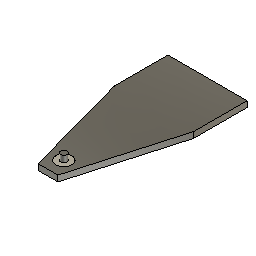
Top Mounting Plate v10 (Autodesk Fusion 360 design; units mm, degrees)
Autodesk Fusion 360 part; units mm, degrees
note: some values were not read from the file. Set by a fixed rule: which sketch regions a step uses.
sketch "Sketch1" plane through (0, 0, 0) normal (0, 0, 1) x (1, 0, 0)
  line L0 (0, 0) -> (-127, 0)
  line L1 (-127, 0) -> (-127, -85.725)
  line L2 (-127, -85.725) -> (0, -85.725)
  line L3 (0, -85.725) -> (0, 0)
  line L4 (-127, -85.725) -> (-80.1138, -255.2229)
  line L5 (0, -85.725) -> (-48.3638, -255.2229)
  line L6 (-80.1138, -255.2229) -> (-48.3638, -255.2229)
  line L7 (-64.2388, -255.2229) -> (-64.2388, -242.5229)
  line L8 (-64.2388, -242.5229) -> (-64.2388, -229.8229)
  circle A0 centre (-64.2388, -229.8229) radius 12.7
  circle A1 centre (-64.2388, -229.8229) radius 5.08
  dimension "d10" = 31.75
  dimension "d11" = 12.7
  dimension "d12" = 12.7
  dimension "d13" = 25.4
  dimension "d14" = 10.16
  dimension "d15" = 127
  dimension "d16" = 85.725
  constraint horizontal L0
  constraint vertical L1
  constraint horizontal L2
  constraint vertical L3
  constraint coincident L0.start L3.end
  constraint horizontal L6
  constraint coincident L4.end L6.start
  constraint coincident L5.end L6.end
  constraint midpoint L6 L7.start
  constraint perpendicular L6 L7
  constraint coincident L8.end A0.centre
  constraint concentric A0 A1
  measures "d10" distance of L4.end L5.end
  measures "d11" distance of L7.start L7.end
  measures "d12" distance of L7.end L8.end
  measures "d13" diameter of A0
  measures "d14" diameter of A1
  measures "d15" distance of L0.start L0.end
  measures "d16" distance of L0.start L2.end
extrude "Extrude1" add sketch "Sketch1" along normal blind 9.525 contours L0 L1 L2 L3 | L2 L4 L5 L6 makes body 1
extrude "Extrude3" add sketch "Sketch1" along normal blind 25 separate body contours A0 makes body 2
extrude "Extrude4" cut 1 faces at (-73.4515, -225.6029, 25) along direction (0, 0, -1) blind 15.475 on bodies 2 bodies 2
extrude "Extrude5" add sketch "Sketch1" along normal blind 20 separate body contours A1 makes body 3
extrude "Extrude6" add sketch "Sketch1" against normal blind 12.7 separate body contours A1 makes body 4
combine "Combine1" operation add target body 3 tool bodies 4
named bodies: "Bearing", "Axle"
